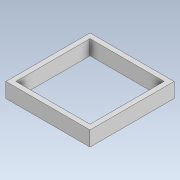
# Autodesk Inventor part: anneau_pack
Saved by Autodesk Inventor 2020 (Build 240168000, 168)
## iProperties
Created: 2020-08-17
Part Number: anneau_pack
Material: Generic
Document SubType Name: Modeling
Designer: Admin
Density: 1 g/cm^3
Appearance: Default
Author: Admin
Autodesk Inventor part; units mm, degrees
ref_plane "YZ Plane" through (0, 0, 0) normal (1, 0, 0) x (0, 1, 0)
ref_plane "XZ Plane" through (0, 0, 0) normal (0, 1, 0) x (-1, 0, 0)
ref_plane "XY Plane" through (0, 0, 0) normal (0, 0, 1) x (1, 0, 0)
sketch "Sketch1" plane through (0, 0, 0) normal (0, 1, 0) x (-1, 0, 0)
  line L0 (0, 0) -> (17, 0)
  line L1 (17, 0) -> (17, -17)
  line L2 (17, -17) -> (0, -17)
  line L3 (0, -17) -> (0, 0)
  line L4 (1, -1) -> (16, -1)
  line L5 (16, -1) -> (16, -16)
  line L6 (16, -16) -> (1, -16)
  line L7 (1, -16) -> (1, -1)
  dimension "d0" = 17
  dimension "d1" = 17
  dimension "d2" = 1
  dimension "d3" = 1
  dimension "d4" = 1
  dimension "d5" = 1
  constraints: 16 end point, 4 parallel, 2 horizontal, 2 perpendicular
  measures "d0" distance of L0.end L1.end
  measures "d1" distance of L1.end L2.end
  measures "d2" distance between parallel lines of L0 L4
  measures "d3" distance between parallel lines of L1 L5
  measures "d4" distance between parallel lines of L3 L7
  measures "d5" distance between parallel lines of L2 L6
extrude "Extrusion1" add sketch "Sketch1" along normal blind 3
body "Solid1"
